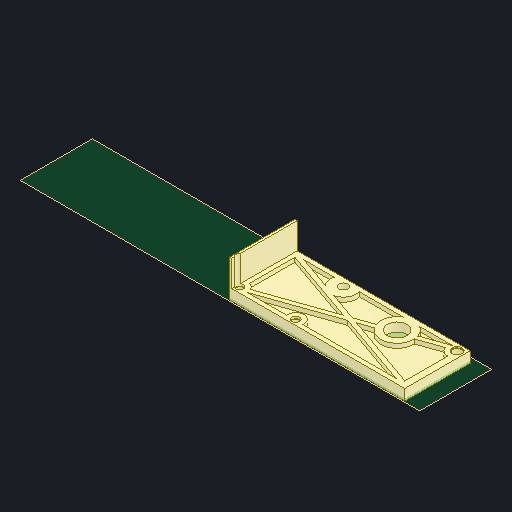
# Autodesk Inventor part: right_gear_holder
Saved by Autodesk Inventor 2023 (Build 270158000, 158)
## iProperties
Created: 2024-04-30
Part Number: right_gear_holder
Material: Nylon 6/6
Document SubType Name: Modeling
Designer: szymo
Density: 1.13 g/cm^3
Appearance: Nylon 6
Mass: 7.32323 g
Surface Area: 88.3576 cm^2
Volume: 6.48073 cm^3
Author: szymo
Autodesk Inventor part; units mm, degrees
ref_plane "YZ Plane" through (0, 0, 0) normal (1, 0, 0) x (0, 1, 0)
ref_plane "XZ Plane" through (0, 0, 0) normal (0, 1, 0) x (-1, 0, 0)
ref_plane "XY Plane" through (0, 0, 0) normal (0, 0, 1) x (1, 0, 0)
ref_plane "Work Plane3" through (-75.5, 11, 0) normal (0, -1, 0) x (1, 0, 0)
sketch "Sketch3" plane through (-75.5, 11, 0) normal (0, -1, 0) x (1, 0, 0)
  line L0 (86.15, 30) -> (166.5, 30) projected
  line L1 (166.5, 0) -> (166.5, 30) projected
  line L2 (116.5, 0) -> (166.5, 0) projected
  line L3 (86.15, 30) -> (86.15, 14.5) projected
  line L4 (86.15, 30) -> (166.5, 30)
  line L5 (166.5, 30) -> (166.5, 0)
  line L6 (166.5, 0) -> (86.15, 0)
  line L7 (86.15, 0) -> (86.15, 30)
  point P0 (75.5, 0)
  constraints: 8 end point, 2 parallel, 1 horizontal, 1 perpendicular
extrude "Extrusion1" add sketch "Sketch3" along normal blind 1
sketch "Sketch4" plane through (-75.5, 11, 0) normal (0, 1, 0) x (1, 0, 0)
  line L0 (86.15, 0) -> (166.5, 0) projected
  line L1 (86.15, -30) -> (86.15, 0) projected
  line L2 (166.5, -30) -> (86.15, -30) projected
  line L3 (166.5, 0) -> (166.5, -30) projected
  circle A0 centre (141.5, -8.5) radius 4.5 projected
  circle A1 centre (111.9101, -3.5563) radius 2 projected
  circle A2 centre (111.9101, -3.5563) radius 6
  line L4 (117.9101, -3.5563) -> (117.9101, 0)
  line L5 (86.15, 0) -> (166.5, 0) projected
  line L6 (105.9101, -3.5563) -> (105.9101, 0)
  point P0 (75.5, 0)
  point P1 (107.0777, 0)
  dimension "d2" = 12
  constraints: 4 end point, 2 point on circle, 2 point on line, 1 centre point, 1 coincident, 1 parallel, 1 perpendicular, 1 tangent
  measures "d2" diameter of A2
extrude "Extrusion2" add sketch "Sketch4" along normal blind 1 contours L0 A2 L6 | L0 A2 | L0 L4 A2 | A1 picked at (111.8297, -0.5236)
sketch "Sketch5" plane through (-75.5, 12, 0) normal (0, 1, 0) x (1, 0, 0)
  line L0 (117.9101, 0) -> (105.9101, 0) projected
  line L1 (105.9101, 0) -> (105.9101, -3.5563) projected
  arc A0 (105.9101, -3.5563) -> (117.9101, -3.5563) centre (111.9101, -3.5563) ccw projected
  line L2 (117.9101, -3.5563) -> (117.9101, 0) projected
  circle A1 centre (111.9101, -3.5563) radius 2 projected
  point P0 (75.5, 0)
extrude "Extrusion3" add sketch "Sketch5" along normal blind 3
sketch "Sketch6" plane through (-75.5, 11, 0) normal (0, 1, 0) x (1, 0, 0)
  circle A0 centre (141.5, -8.5) radius 4.5 projected
  circle A1 centre (141.5, -8.5) radius 8.5
  line L0 (150, -8.5) -> (149.6698, 0)
  line L1 (86.15, 0) -> (166.5, 0) projected
  line L2 (133, -8.5) -> (133, 0)
  line L3 (117.9101, 0) -> (166.5, 0) projected
  point P0 (75.5, 0)
  dimension "d7" = 17
  constraints: 4 end point, 2 point on circle, 2 point on line, 1 centre point, 1 coincident, 1 vertical
  measures "d7" diameter of A1
ref_plane "Work Plane4" through (60.3074, 16, 2.8074) normal (0, -1, 0) x (0.988717, 0, 0.1497953)
extrude "Extrusion4" add sketch "Sketch6" along normal blind 4 contours A1 L0 | L2 L1 A1 | L1 L0 A1 picked at (148.4648, -7.0125)
sketch "Sketch7" plane through (-75.5, 11, 0) normal (0, 1, 0) x (1, 0, 0)
  line L0 (166.5, -30) -> (86.15, -30) projected
  line L1 (166.5, 0) -> (166.5, -30) projected
  line L2 (86.15, -30) -> (86.15, 0) projected
  line L3 (86.15, 0) -> (105.9101, 0) projected
  line L4 (105.9101, 0) -> (105.9101, -3.5563) projected
  arc A0 (105.9101, -3.5563) -> (117.9101, -3.5563) centre (111.9101, -3.5563) ccw projected
  line L5 (117.9101, -3.5563) -> (117.9101, 0) projected
  line L6 (117.9101, 0) -> (105.9101, 0) projected
  circle A1 centre (111.9101, -3.5563) radius 2 projected
  line L7 (149.6698, 0) -> (133, 0) projected
  line L8 (133, 0) -> (133, -8.5) projected
  arc A2 (133, -8.5) -> (150, -8.5) centre (141.5, -8.5) ccw projected
  line L9 (150, -8.5) -> (149.6698, 0) projected
  circle A3 centre (141.5, -8.5) radius 4.5 projected
  line L10 (149.6698, 0) -> (166.5, 0) projected
  line L11 (117.9101, 0) -> (133, 0) projected
  point P0 (75.5, 0)
extrude "Extrusion5" add sketch "Sketch7" along normal blind 4 contours L0 L2 L3 L4 A0 L5 L11 L8 A2 L9 L10 L1
sketch "Sketch8" plane through (-75.5, 15, 0) normal (0, 1, 0) x (1, 0, 0)
  circle A0 centre (114, -27.5) radius 1.55 projected
  circle A1 centre (88.25, -27.5) radius 1.55 projected
  point P0 (75.5, 0)
  constraints: 2 coincident
hole "Hole1" at (12.75, 15, 27.5) at (38.5, 15, 27.5) direction (0, -1, 0) diameter 3 depth 4 counterbore diameter 3.5 counterbore depth 1
sketch "Sketch9" plane through (-75.5, 15, 0) normal (0, 1, 0) x (1, 0, 0)
  circle A0 centre (163.5, -3) radius 1.8 projected
  point P0 (75.5, 0)
hole "Hole2" at (88, 15, 3) direction (0, -1, 0) diameter 4 depth 4.5 counterbore diameter 4.6 counterbore depth 0.5
sketch "Sketch10" plane through (10.65, 10, 0) normal (-1, 0, 0) x (0, 0, 1)
  line L0 (0, 0) -> (0, 5) projected
  line L1 (30, 0) -> (0, 0) projected
  line L2 (30, 5) -> (30, 0) projected
  line L3 (0, 5) -> (30, 5) projected
  line L4 (0, 17) -> (30, 17) projected
  line L5 (0, 5) -> (30, 5)
  line L6 (30, 5) -> (30, 17)
  line L7 (30, 17) -> (0, 17)
  line L8 (0, 17) -> (0, 5)
  point P0 (0, -10)
  constraints: 8 end point, 2 parallel, 1 horizontal, 1 perpendicular
extrude "Extrusion6" add sketch "Sketch10" against normal blind 1 contours L8 L4 L6 L3
sketch "Sketch11" plane through (10.65, 27, 30) normal (0, 1, 0) x (1, 0, 0)
  arc A0 (1, 1.1389) -> (1, 3.8611) centre (2.1, 2.5) ccw projected
  circle A1 centre (2.1, 2.5) radius 1.75
  point P0 (-10.65, 30)
  constraints: 1 centre point, 1 coincident, 1 concentric
extrude "Extrusion7" cut sketch "Sketch11" against normal up to surface (13 mm away)
sketch "Sketch12" plane through (-75.5, 15, 0) normal (0, 1, 0) x (1, 0, 0)
  circle A0 centre (141.5, -8.5) radius 4.5 projected
  circle A1 centre (111.9101, -3.5563) radius 2 projected
  circle A2 centre (114, -27.5) radius 1.75 projected
  circle A3 centre (163.5, -3) radius 2.3 projected
  line L0 (87.15, 0) -> (87.15, -26.1389) projected
  arc A4 (87.15, -28.8611) -> (87.15, -26.1389) centre (88.25, -27.5) ccw projected
  line L1 (87.15, -28.8611) -> (87.15, -30) projected
  line L2 (87.15, -30) -> (166.5, -30) projected
  line L3 (166.5, -30) -> (166.5, 0) projected
  line L4 (166.5, 0) -> (87.15, 0) projected
  circle A5 centre (141.5, -8.5) radius 7.5
  circle A6 centre (111.9101, -3.5563) radius 6
  circle A7 centre (163.5, -3) radius 4.3
  circle A8 centre (114, -27.5) radius 1.75 projected
  circle A9 centre (114, -27.5) radius 3.75
  circle A10 centre (88.25, -27.5) radius 1.5 projected
  circle A11 centre (88.25, -27.5) radius 3.75
  line L5 (89.15, -30) -> (89.15, 0)
  line L6 (86.15, 0) -> (166.5, 0) projected
  line L7 (163.5, -30) -> (163.5, 0)
  line L8 (86.15, -30) -> (86.15, 0) projected
  line L9 (163.5, -28) -> (89.15, -28)
  line L10 (89.15, -2) -> (163.5, -2)
  line L11 (163.5, -2) -> (89.15, -28) construction
  line L12 (89.15, -2) -> (163.5, -28) construction
  line L13 (163.5, -26.9406) -> (92.1794, -2)
  line L14 (89.15, -3.0594) -> (160.4706, -28)
  line L15 (163.5, -3.0594) -> (92.1794, -28)
  line L16 (160.4706, -2) -> (89.15, -26.9406)
  point P0 (75.5, 0)
  point P1 (91.7069, -26.0465)
  point P2 (123.2956, -15)
  point P3 (89.15, -23.8596)
  point P4 (126.325, -16.0594)
  point P5 (110.2835, -28)
  point P6 (117.7165, -28)
  point P7 (148.6203, -6.144)
  point P8 (159.2378, -2.4311)
  point P9 (159.3179, -2)
  point P10 (145.2417, -2)
  point P11 (126.325, -13.9406)
  point P12 (134.4631, -11.0947)
  point P13 (117.7048, -2)
  point P14 (106.1155, -2)
  point P15 (135.4128, -12.8814)
  point P16 (129.3544, -15)
  point P17 (163.5, -7.3)
  point P18 (159.4599, -4.4722)
  point P19 (148.991, -8.1331)
  point P20 (137.7583, -2)
  point P21 (113.1662, -2)
  point P22 (110.654, -2)
  point P23 (107.1779, -7.2449)
  point P24 (113.3124, -9.3902)
  dimension "d30" = 3.5
  dimension "d31" = 1.75
  dimension "d32" = 4
  dimension "d33" = 9
  dimension "d34" = 4.6
  dimension "d35" = 7.5
  dimension "d36" = 7.5
  dimension "d37" = 12
  dimension "d38" = 15
  dimension "d39" = 8.6
  dimension "d40" = 2
  dimension "d41" = 3
  dimension "d42" = 2
  dimension "d43" = 3
  dimension "d44" = 1
  dimension "d45" = 1
  dimension "d46" = 1
  dimension "d47" = 1
  constraints: 20 end point, 16 point on line, 7 parallel, 5 centre point, 5 coincident, 2 perpendicular
  measures "d30" diameter of A2
  measures "d31" radius of A4
  measures "d32" diameter of A1
  measures "d33" diameter of A0
  measures "d34" diameter of A3
  measures "d35" diameter of A11
  measures "d36" diameter of A9
  measures "d37" diameter of A6
  measures "d38" diameter of A5
  measures "d39" diameter of A7
  measures "d40" distance between parallel lines of L2 L9
  measures "d41" distance between parallel lines of L8 L5
  measures "d42" distance between parallel lines of L6 L10
  measures "d43" distance between parallel lines of L3 L7
  measures "d44" distance between parallel lines of L11 L16
  measures "d45" distance between parallel lines of L15 L11
  measures "d46" distance between parallel lines of L12 L14
  measures "d47" distance between parallel lines of L12 L13
extrude "Extrusion8" cut sketch "Sketch12" against normal blind 2 contours A5 L10 A7 L16 | L15 A7 L7 L13 A5 | L16 L13 A6 L10 A5 | A7 L10 L16 | L16 A11 L5 L14 | L14 L9 A9 L15 | A1 L10 | L13 L10 A6 picked at (112.1123, -3.2836)
sketch "Sketch13" plane through (-75.5, 10, 0) normal (0, -1, 0) x (1, 0, 0)
  line L0 (89.15, 23.8596) -> (89.15, 3.0594) projected
  line L1 (89.15, 3.0594) -> (123.2956, 15) projected
  line L2 (123.2956, 15) -> (91.7069, 26.0465) projected
  arc A0 (89.15, 23.8596) -> (91.7069, 26.0465) centre (88.25, 27.5) ccw projected
  arc A1 (145.2417, 2) -> (148.6203, 6.144) centre (141.5, 8.5) ccw projected
  line L3 (145.2417, 2) -> (160.4706, 2) projected
  line L4 (160.4706, 2) -> (148.6203, 6.144) projected
  line L5 (92.1794, 2) -> (106.1155, 2) projected
  arc A2 (107.1779, 7.2449) -> (106.1155, 2) centre (111.9101, 3.5563) ccw projected
  line L6 (107.1779, 7.2449) -> (92.1794, 2) projected
  arc A3 (110.2835, 28) -> (117.7165, 28) centre (114, 27.5) ccw projected
  line L7 (110.2835, 28) -> (92.1794, 28) projected
  line L8 (92.1794, 28) -> (126.325, 16.0594) projected
  line L9 (126.325, 16.0594) -> (160.4706, 28) projected
  line L10 (160.4706, 28) -> (117.7165, 28) projected
  line L11 (163.5, 7.3) -> (163.5, 26.9406) projected
  line L12 (163.5, 26.9406) -> (129.3544, 15) projected
  line L13 (129.3544, 15) -> (135.4128, 12.8814) projected
  arc A4 (148.991, 8.1331) -> (135.4128, 12.8814) centre (141.5, 8.5) ccw projected
  line L14 (148.991, 8.1331) -> (159.4599, 4.4722) projected
  arc A5 (163.5, 7.3) -> (159.4599, 4.4722) centre (163.5, 3) ccw projected
  line L15 (117.7048, 2) -> (137.7583, 2) projected
  arc A6 (134.4631, 11.0947) -> (137.7583, 2) centre (141.5, 8.5) ccw projected
  line L16 (134.4631, 11.0947) -> (126.325, 13.9406) projected
  line L17 (126.325, 13.9406) -> (113.3124, 9.3902) projected
  arc A7 (117.7048, 2) -> (113.3124, 9.3902) centre (111.9101, 3.5563) ccw projected
  circle A8 centre (141.5, 8.5) radius 4.5 projected
  circle A9 centre (111.9101, 3.5563) radius 2 projected
  circle A10 centre (114, 27.5) radius 1.75 projected
  circle A11 centre (163.5, 3) radius 2.3 projected
  line L18 (87.15, 0) -> (87.15, 26.1389) projected
  arc A12 (87.15, 26.1389) -> (87.15, 28.8611) centre (88.25, 27.5) ccw projected
  line L19 (87.15, 28.8611) -> (87.15, 30) projected
  line L20 (87.15, 30) -> (166.5, 30) projected
  line L21 (166.5, 30) -> (166.5, 0) projected
  line L22 (166.5, 0) -> (87.15, 0) projected
  point P0 (75.5, 0)
extrude "Extrusion9" cut sketch "Sketch13" against normal blind 2 contours A0 L2 L1 L0 | A1 L4 L3 | L6 A2 L5 | A3 L10 L9 L8 L7 | A5 L14 A4 L13 L12 L11 | A7 L17 L16 A6 L15
equation "\"d45\" = d44"
equation "\"d47\" = d46"
body "Solid1"
